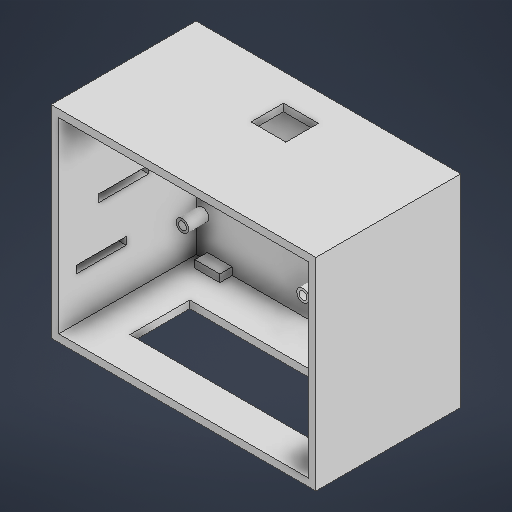
# Autodesk Inventor part: air-monitor_enclosure
Saved by Autodesk Inventor 2026.1 (Build 301233020, 233B)
## iProperties
Created: 2026-06-10
Part Number: air-monitor_enclosure
Material: Generic
Document SubType Name: Modeling
Designer: astro
Density: 1 g/cm^3
Appearance: Default
Author: astro
Autodesk Inventor part; units mm, degrees
ref_plane "YZ Plane" through (0, 0, 0) normal (1, 0, 0) x (0, 1, 0)
ref_plane "XZ Plane" through (0, 0, 0) normal (0, 1, 0) x (-1, 0, 0)
ref_plane "XY Plane" through (0, 0, 0) normal (0, 0, 1) x (1, 0, 0)
sketch "Sketch1" plane through (0, 0, 0) normal (0, 0, 1) x (1, 0, 0)
  line L0 (0, 0) -> (106, 0)
  line L1 (106, 0) -> (106, 81)
  line L2 (106, 81) -> (0, 81)
  line L3 (0, 81) -> (0, 0)
  dimension "d0" = 106
  dimension "d1" = 81
  constraints: 8 end point, 2 parallel, 1 horizontal, 1 perpendicular
  measures "d0" distance of L2.end L1.end
  measures "d1" distance of L1.end L0.end
extrude "Extrusion1" add sketch "Sketch1" along normal blind 58
shell "Shell1" thickness 3 removed faces 1 at (70.6667, 27, 58)
sketch "Sketch2" plane through (0, 0, 0) normal (0, -1, 0) x (1, 0, 0)
  line L0 (17.5, 20) -> (88.5, 20)
  line L1 (88.5, 20) -> (88.5, 44)
  line L2 (88.5, 44) -> (17.5, 44)
  line L3 (17.5, 44) -> (17.5, 20)
  line L4 (0, 0) -> (0, 58) projected
  line L5 (0, 0) -> (106, 0) projected
  dimension "d5" = 71
  dimension "d6" = 24
  dimension "d7" = 17.5
  dimension "d8" = 20
  constraints: 8 end point, 2 parallel, 1 horizontal, 1 perpendicular
  measures "d5" distance of L2.end L1.end
  measures "d6" distance of L1.end L0.end
  measures "d7" distance between parallel lines of L3 L4
  measures "d8" distance between parallel lines of L5 L0
extrude "Extrusion2" cut sketch "Sketch2" against normal blind 3
sketch "Sketch3" plane through (0, 81, 0) normal (0, 1, 0) x (1, 0, 0)
  line L0 (60, -24) -> (46, -24)
  line L1 (46, -24) -> (46, -11)
  line L2 (46, -11) -> (60, -11)
  line L3 (60, -11) -> (60, -24)
  line L4 (106, 0) -> (106, -58) projected
  line L5 (106, 0) -> (0, 0) projected
  dimension "d11" = 14
  dimension "d12" = 13
  dimension "d13" = 46
  dimension "d14" = 11
  constraints: 8 end point, 2 parallel, 1 horizontal, 1 perpendicular
  measures "d11" distance of L1.end L2.end
  measures "d12" distance of L0.end L1.end
  measures "d13" distance between parallel lines of L3 L4
  measures "d14" distance between parallel lines of L5 L2
extrude "Extrusion3" cut sketch "Sketch3" against normal blind 3
sketch "Sketch4" plane through (0, 0, 0) normal (-1, 0, 0) x (0, 0, 1)
  line L0 (33, 63.75) -> (13, 63.75)
  line L1 (13, 63.75) -> (13, 60.75)
  line L2 (13, 60.75) -> (33, 60.75)
  line L3 (33, 60.75) -> (33, 63.75)
  line L4 (42, 43.5) -> (22, 43.5)
  line L5 (22, 43.5) -> (22, 40.5)
  line L6 (22, 40.5) -> (42, 40.5)
  line L7 (42, 40.5) -> (42, 43.5)
  line L8 (31, 23.25) -> (51, 23.25)
  line L9 (51, 23.25) -> (51, 20.25)
  line L10 (51, 20.25) -> (31, 20.25)
  line L11 (31, 20.25) -> (31, 23.25)
  line L12 (0, 81) -> (0, 0) projected
  line L13 (0, 81) -> (58, 81) projected
  line L14 (0, 0) -> (58, 0) projected
  dimension "d17" = 20
  dimension "d18" = 3
  dimension "d19" = 20
  dimension "d20" = 3
  dimension "d21" = 20
  dimension "d22" = 3
  dimension "d23" = 13
  dimension "d24" = 22
  dimension "d25" = 31
  dimension "d90" = 20.25
  dimension "d91" = 40.5
  dimension "d92" = 60.75
  constraints: 24 end point, 6 parallel, 3 horizontal, 3 perpendicular
  measures "d17" distance of L2.end L1.end
  measures "d18" distance of L1.end L0.end
  measures "d19" distance of L6.end L5.end
  measures "d20" distance of L5.end L4.end
  measures "d21" distance of L9.end L10.end
  measures "d22" distance of L8.end L9.end
  measures "d23" distance between parallel lines of L12 L1
  measures "d24" distance between parallel lines of L12 L5
  measures "d25" distance between parallel lines of L12 L11
  measures "d90" distance between parallel lines of L14 L10
  measures "d91" distance between parallel lines of L14 L6
  measures "d92" distance between parallel lines of L14 L2
sketch "Sketch5" plane through (3, 78, 3) normal (0, 0, 1) x (1, 0, 0)
  circle A0 centre (2.54, -59.76) radius 2.5
  line L0 (0, 0) -> (0, -75) projected
  line L1 (0, -75) -> (100, -75) projected
  circle A1 centre (2.54, -8.96) radius 2.5
  circle A2 centre (50.8, -8.96) radius 2.5
  circle A3 centre (50.8, -59.76) radius 2.5
  point P0 (-3, -78)
  dimension "d28" = 5
  dimension "d29" = 2.54
  dimension "d30" = 15.24
  dimension "d31" = 5
  dimension "d32" = 2.54
  dimension "d33" = 66.04
  dimension "d34" = 5
  dimension "d35" = 50.8
  dimension "d36" = 66.04
  dimension "d37" = 5
  dimension "d38" = 50.8
  dimension "d39" = 15.24
  constraints: 4 centre point
  measures "d28" diameter of A0
  measures "d29" distance from line of L0 A0.centre
  measures "d30" distance from line of L1 A0.centre
  measures "d31" diameter of A1
  measures "d32" distance from line of L0 A1.centre
  measures "d33" distance from line of L1 A1.centre
  measures "d34" diameter of A2
  measures "d35" distance from line of L0 A2.centre
  measures "d36" distance from line of A2.centre L1
  measures "d37" diameter of A3
  measures "d38" distance from line of L0 A3.centre
  measures "d39" distance from line of L1 A3.centre
extrude "Extrusion4" add sketch "Sketch5" along normal blind 8
sketch "Sketch6" plane through (5.54, 69.04, 11) normal (0, 0, 1) x (1, 0, 0)
  point P0 (-5.54, -69.04)
  point P1 (0, 0)
sketch "Sketch7" plane through (5.54, 18.24, 11) normal (0, 0, 1) x (1, 0, 0)
  circle A0 centre (48.26, 0) radius 2.5 projected
  point P0 (-5.54, -18.24)
  point P1 (0, 0)
  constraints: 1 coincident
sketch "Sketch8" plane through (53.8, 69.04, 11) normal (0, 0, 1) x (1, 0, 0)
  point P0 (-53.8, -69.04)
  point P1 (0, 0)
hole "Hole1" at (5.54, 69.04, 11) direction (0, 0, -1) diameter 3.2 depth 8
hole "Hole2" at (53.8, 69.04, 11) direction (0, 0, -1) diameter 3.2 depth 8
hole "Hole3" at (5.54, 18.24, 11) direction (0, 0, -1) diameter 3.2 depth 8
sketch "Sketch9" plane through (53.8, 18.24, 11) normal (0, 0, 1) x (1, 0, 0)
  point P0 (-53.8, -18.24)
  point P1 (0, 0)
hole "Hole4" at (53.8, 18.24, 11) direction (0, 0, -1) diameter 3.2 depth 8
sketch "Sketch10" plane through (3, 3, 3) normal (0, 1, 0) x (1, 0, 0)
  line L0 (85.5, -5) -> (95.5, -5)
  line L1 (95.5, -5) -> (95.5, 0)
  line L2 (95.5, 0) -> (85.5, 0)
  line L3 (85.5, 0) -> (85.5, -5)
  line L4 (85.5, -17) -> (85.5, -41) projected
  line L5 (0, 0) -> (100, 0) projected
  line L6 (14.5, -5) -> (4.5, -5)
  line L7 (4.5, -5) -> (4.5, 0)
  line L8 (4.5, 0) -> (14.5, 0)
  line L9 (14.5, 0) -> (14.5, -5)
  line L10 (14.5, -41) -> (14.5, -17) projected
  point P0 (-3, 3)
  dimension "d70" = 10
  dimension "d71" = 5
  dimension "d72" = 0
  dimension "d74" = 10
  dimension "d75" = 5
  dimension "d76" = 0
  dimension "d77" = 0
  dimension "d80" = 0
  constraints: 16 end point, 4 parallel, 2 horizontal, 2 perpendicular
  measures "d70" distance of L2.end L1.end
  measures "d71" distance of L1.end L0.end
  measures "d72" distance between parallel lines of L4 L3
  measures "d74" distance of L7.end L8.end
  measures "d75" distance of L6.end L7.end
  measures "d76" distance between parallel lines of L10 L9
  measures "d77" distance between parallel lines of L5 L8
  measures "d80" distance between parallel lines of L5 L2
extrude "Extrusion5" add sketch "Sketch10" along normal blind 3
sketch "Sketch11" plane through (0, 0, 0) normal (0, 0, -1) x (-1, 0, 0)
  circle A0 centre (-53, 58) radius 5
  circle A1 centre (-53, 23) radius 5
  line L0 (-106, 0) -> (-106, 81) projected
  line L1 (-106, 81) -> (0, 81) projected
  line L2 (0, 0) -> (-106, 0) projected
  dimension "d81" = 10
  dimension "d82" = 10
  dimension "d83" = 53
  dimension "d84" = 53
  dimension "d85" = 23
  dimension "d86" = 23
  constraints: 2 centre point
  measures "d81" diameter of A0
  measures "d82" diameter of A1
  measures "d83" distance from line of L0 A0.centre
  measures "d84" distance from line of L0 A1.centre
  measures "d85" distance from line of L1 A0.centre
  measures "d86" distance from line of L2 A1.centre
extrude "Extrusion6" cut sketch "Sketch11" against normal blind 3.5
extrude "Extrusion7" cut sketch "Sketch4" against normal blind 3.5
body "Solid1"
